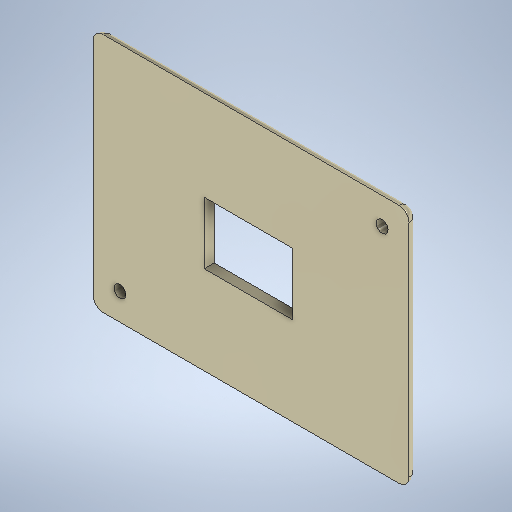
# Autodesk Inventor part: limb_cover
Saved by Autodesk Inventor 2025 (Build 290162000, 162)
## iProperties
Created: 2026-06-03
Part Number: limb_cover
Material: Generic
Document SubType Name: Modeling
Designer: rohan
Density: 1 g/cm^3
Appearance: 1.5in Square - Medium Blue
Author: rohan
Autodesk Inventor part; units mm, degrees
ref_plane "YZ Plane" through (0, 0, 0) normal (1, 0, 0) x (0, 1, 0)
ref_plane "XZ Plane" through (0, 0, 0) normal (0, 1, 0) x (-1, 0, 0)
ref_plane "XY Plane" through (0, 0, 0) normal (0, 0, 1) x (1, 0, 0)
sketch "Sketch1" plane through (0, 0, 0) normal (0, 0, 1) x (1, 0, 0)
  line L0 (-19.8753, 2.5645) -> (43.3247, 2.5645)
  line L1 (43.3247, 2.5645) -> (43.3247, -45.6355)
  line L2 (43.3247, -45.6355) -> (-19.8753, -45.6355)
  line L3 (-19.8753, -45.6355) -> (-19.8753, 2.5645)
  circle A0 centre (37.9747, -2.7855) radius 2.1
  circle A1 centre (-14.5253, -40.2855) radius 2.1
  circle A2 centre (37.9747, -2.7855) radius 1.2
  circle A3 centre (-14.5253, -40.2855) radius 1.2
  point P0 (0, 0)
  dimension "d0" = 63.2
  dimension "d1" = 48.2
  dimension "d6" = 4.2
  dimension "d7" = 4.2
  dimension "d8" = 5.35
  dimension "d9" = 5.35
  dimension "d10" = 5.35
  dimension "d11" = 5.35
  dimension "d12" = 2.4
  dimension "d13" = 2.4
  constraints: 8 end point, 4 centre point, 2 coincident, 2 parallel, 1 horizontal, 1 perpendicular
  measures "d0" distance of L1.end L2.end
  measures "d1" distance of L0.end L1.end
  measures "d6" diameter of A0
  measures "d7" diameter of A1
  measures "d8" distance from line of A0.centre L0
  measures "d9" distance from line of L1 A0.centre
  measures "d10" distance from line of L3 A1.centre
  measures "d11" distance from line of L2 A1.centre
  measures "d12" diameter of A2
  measures "d13" diameter of A3
extrude "Extrusion1" add sketch "Sketch1" along normal blind 2 contours L0 L1 L2 L3 | A0 | A1 | A2 | A3
fillet "Fillet1" radius 2 2 edges at (-19.8753, 2.5645, 1) (-19.8753, -45.6355, 1)
fillet "Fillet2" radius 2 2 edges at (43.3247, 2.5645, 1) (43.3247, -45.6355, 1)
sketch "Sketch2" plane through (0, 0, 0) normal (0, 0, -1) x (-1, 0, 0)
  circle A0 centre (14.5253, -40.2855) radius 2.1
  circle A1 centre (-37.9747, -2.7855) radius 2.1
  circle A2 centre (14.5253, -40.2855) radius 1.2
  circle A3 centre (-37.9747, -2.7855) radius 1.2
  line L0 (17.8753, -45.6355) -> (-41.3247, -45.6355) projected
  line L1 (19.8753, 0.5645) -> (19.8753, -43.6355) projected
  line L2 (-43.3247, -43.6355) -> (-43.3247, 0.5645) projected
  line L3 (-41.3247, 2.5645) -> (17.8753, 2.5645) projected
  point P0 (0, 0)
  dimension "d14" = 4.2
  dimension "d15" = 4.2
  dimension "d16" = 2.4
  dimension "d17" = 2.4
  dimension "d18" = 5.35
  dimension "d19" = 5.35
  dimension "d20" = 5.35
  dimension "d21" = 5.35
  constraints: 4 centre point, 2 coincident
  measures "d14" diameter of A0
  measures "d15" diameter of A1
  measures "d16" diameter of A2
  measures "d17" diameter of A3
  measures "d18" distance from line of A0.centre L0
  measures "d19" distance from line of A0.centre L1
  measures "d20" distance from line of L2 A1.centre
  measures "d21" distance from line of L3 A1.centre
extrude "Extrusion3" cut sketch "Sketch2" against normal blind 2.2 contours A2 | A3
fillet "Fillet3" radius 2 8 edges at (42.7389, -45.0497, 0) (43.3247, -21.5355, 0) (42.7389, 1.9787, 0) (11.7247, 2.5645, 0) (-19.2896, 1.9787, 0) (-19.8753, -21.5355, 0) (-19.2896, -45.0497, 0) (11.7247, -45.6355, 0)
sketch "Sketch4" plane through (0, 0, 0) normal (0, 0, -1) x (-1, 0, 0)
  line L0 (-2.3639, -27.9277) -> (-20.0539, -27.9277)
  line L1 (-20.0539, -27.9277) -> (-20.0539, -15.5277)
  line L2 (-20.0539, -15.5277) -> (-2.3639, -15.5277)
  line L3 (-2.3639, -15.5277) -> (-2.3639, -27.9277)
  point P0 (0, 0)
  dimension "d27" = 17.69
  dimension "d28" = 12.4
  constraints: 8 end point, 2 parallel, 1 horizontal, 1 perpendicular
  measures "d27" distance of L1.end L2.end
  measures "d28" distance of L0.end L1.end
extrude "Extrusion4" cut sketch "Sketch4" against normal blind 2.2
body "Solid1"
